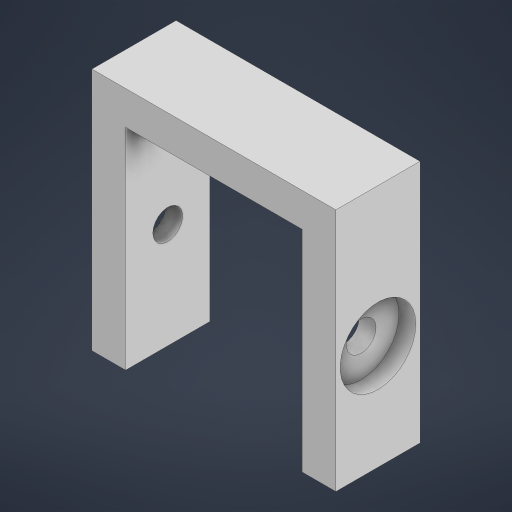
# Autodesk Inventor part: Inner_Tube_Endcap2
Saved by Autodesk Inventor 2023 (Build 270158000, 158)
## iProperties
Created: 2024-02-22
Part Number: Inner_Tube_Endcap2
Material: Generic
Document SubType Name: Modeling
Designer: kelle
Density: 1 g/cm^3
Appearance: Default
Author: kelle
Autodesk Inventor part; units mm, degrees
ref_plane "YZ Plane" through (0, 0, 0) normal (1, 0, 0) x (0, 1, 0)
ref_plane "XZ Plane" through (0, 0, 0) normal (0, 1, 0) x (-1, 0, 0)
ref_plane "XY Plane" through (0, 0, 0) normal (0, 0, 1) x (1, 0, 0)
sketch "Sketch1" plane through (0, 0, 0) normal (0, 0, 1) x (1, 0, 0)
  line L0 (13.335, -13.335) -> (-13.335, -13.335) construction
  line L1 (-13.335, -13.335) -> (-13.335, 13.335)
  line L2 (-13.335, 13.335) -> (13.335, 13.335)
  line L3 (13.335, 13.335) -> (13.335, -13.335)
  line L4 (13.335, -13.335) -> (-13.335, 13.335) construction
  line L5 (-13.335, -13.335) -> (13.335, 13.335) construction
  line L6 (18.415, 18.415) -> (-18.415, 18.415)
  line L7 (-18.415, 18.415) -> (-18.415, -18.415)
  line L8 (-18.415, -18.415) -> (18.415, -18.415)
  line L9 (18.415, -18.415) -> (18.415, 18.415)
  line L10 (-13.335, -13.335) -> (-13.335, -18.415)
  line L11 (13.335, -13.335) -> (13.335, -18.415)
  point P0 (0, 0)
  dimension "d0" = 26.67
  dimension "d1" = 26.67
  dimension "d2" = 5.08
  constraints: 24 end point, 4 parallel, 4 perpendicular, 2 midpoint, 2 point on line, 1 horizontal, 3 other
  measures "d0" distance of L1.end L2.end
  measures "d1" distance of L0.end L1.end
  measures "d2" distance between parallel lines of L2 L6
extrude "Extrusion1" add sketch "Sketch1" along normal blind 12.7 contours L10 L8 L7 L6 L9 L11 L3 L2 L1
sketch "Sketch2" plane through (18.415, -18.415, 0) normal (1, 0, 0) x (0, 0, -1)
  line L0 (0, 0) -> (0, 36.83) projected
  line L1 (0, 36.83) -> (-12.7, 36.83) projected
  line L2 (-12.7, 0) -> (-12.7, 36.83) projected
  line L3 (0, 0) -> (-12.7, 0) projected
  line L4 (0, 36.83) -> (-12.7, 36.83) construction
  line L5 (-6.35, 36.83) -> (-6.35, 0) construction
  line L6 (0, 0) -> (-12.7, 0) construction
  line L7 (0, 31.75) -> (-12.7, 31.75) construction
  line L8 (-12.7, 0) -> (-12.7, 31.75) construction
  line L9 (-12.7, 15.875) -> (0, 15.875) construction
  line L10 (0, 0) -> (0, 31.75) construction
  circle A0 centre (-6.35, 15.875) radius 2.25
  circle A1 centre (-6.35, 15.875) radius 5.715
  point P0 (0, 18.415)
  dimension "d5" = 4.5
  dimension "d6" = 11.43
  constraints: 5 midpoint, 4 end point, 2 centre point, 1 coincident
  measures "d5" diameter of A0
  measures "d6" diameter of A1
extrude "Extrusion2" cut sketch "Sketch2" against normal through all contours A0
extrude "Extrusion3" cut sketch "Sketch2" against normal blind 2.54 contours A1
sketch "Sketch3" plane through (-18.415, -18.415, 0) normal (-1, 0, 0) x (0, 0, 1)
  circle A0 centre (6.35, 15.875) radius 2.25 projected
  circle A1 centre (6.35, 15.875) radius 5.715
  point P0 (0, 18.415)
  dimension "d11" = 11.43
  constraints: 1 centre point, 1 coincident
  measures "d11" diameter of A1
extrude "Extrusion4" cut sketch "Sketch3" against normal blind 2.54
body "Solid1"
